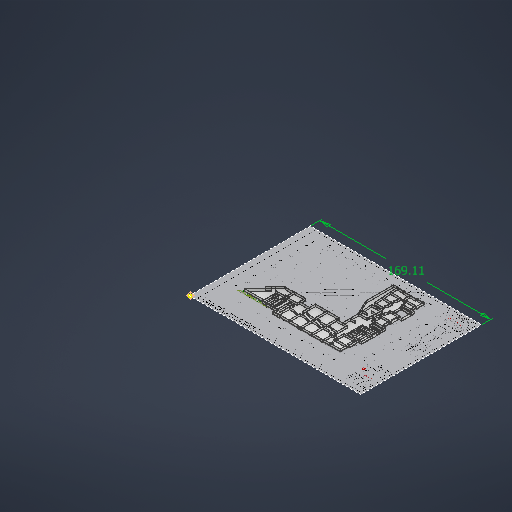
# Autodesk Inventor part: floor-6
Saved by Autodesk Inventor 2026.1 (Build 301233000, 233)
## iProperties
Created: 2025-07-25
Part Number: floor-6
Material: Generic
Document SubType Name: Modeling
Designer: diego
Density: 1 g/cm^3
Appearance: Default
Author: diego
Autodesk Inventor part; units mm, degrees
ref_plane "YZ Plane" through (0, 0, 0) normal (1, 0, 0) x (0, 1, 0)
ref_plane "XZ Plane" through (0, 0, 0) normal (0, 1, 0) x (-1, 0, 0)
ref_plane "XY Plane" through (0, 0, 0) normal (0, 0, 1) x (1, 0, 0)
sketch "Sketch1" plane through (0, 0, 0) normal (0, 1, 0) x (-1, 0, 0)
  line L0 (-169110.0554, 0) -> (0, 0) construction
  line L1 (0, 0) -> (0, -119446.8965) construction
  line L2 (0, -119446.8965) -> (-169110.0554, -119446.8965) construction
  line L3 (-169110.0554, -119446.8965) -> (-169110.0554, 0) construction
  dimension "d10" = 169110.0554
  constraints: 1 coincident, 1 horizontal, 2 other
  measures "d10" distance of L1.end L2.end
sketch "Sketch2" plane through (0, 0, 0) normal (0, 1, 0) x (-1, 0, 0)
  line L0 (-42513, -43975) -> (-42513, -44536)
  line L1 (-42513, -44536) -> (-40080, -44536)
  line L2 (-40080, -44536) -> (-36578.0094, -48027.3226)
  line L3 (-36484.618, -48120.4296) -> (-41280.5342, -52931)
  line L4 (-49108, -44536) -> (-42818, -44536)
  line L5 (-42818, -44536) -> (-42818, -43975)
  line L6 (-42818, -43975) -> (-42513, -43975)
  line L7 (-41376.4054, -52704.3063) -> (-36821.5408, -48135.524)
  line L8 (-36821.5408, -48135.524) -> (-40203.6055, -44763.7619)
  line L9 (-40203.6055, -44763.7619) -> (-42568, -44763.7619)
  line L10 (-42568, -44763.7619) -> (-49108, -44763.7619)
  line L11 (-49108, -44763.7619) -> (-49108, -44536)
  line L12 (-42513, -42019.3536) -> (-42818, -42019.3536)
  line L13 (-42818, -42019.3536) -> (-42818, -41767)
  line L14 (-42818, -41767) -> (-46373, -41767)
  line L15 (-46373, -41767) -> (-46373, -39722)
  line L16 (-46373, -39722) -> (-46111.7717, -39722)
  line L17 (-46111.7717, -39722) -> (-46111.7717, -41553)
  line L18 (-46111.7717, -41553) -> (-42818, -41553)
  line L19 (-42818, -41553) -> (-42818, -39965)
  line L20 (-42818, -39965) -> (-45192, -39965)
  line L21 (-45192, -39965) -> (-45192, -39722)
  line L22 (-45192, -39722) -> (-42818, -39722)
  line L23 (-42513, -29103) -> (-57094, -29103)
  line L24 (-42818, -39722) -> (-42818, -29418.9509)
  line L25 (-42818, -29418.9509) -> (-46077.2284, -29418.9509)
  line L26 (-46077.2284, -29418.9509) -> (-46077.2284, -37968.9509)
  line L27 (-46077.2284, -37968.9509) -> (-44184.9712, -37968.9509)
  line L28 (-44184.9712, -37968.9509) -> (-44184.9712, -38782.9509)
  line L29 (-44184.9712, -38782.9509) -> (-44428.549, -38782.9509)
  line L30 (-44428.549, -38782.9509) -> (-44428.549, -38197.9509)
  line L31 (-44428.549, -38197.9509) -> (-48923.6909, -38197.9509)
  line L32 (-48923.6909, -38197.9509) -> (-48923.6909, -37968.9509)
  line L33 (-48923.6909, -37968.9509) -> (-46371.8628, -37968.9509)
  line L34 (-46371.8628, -37968.9509) -> (-46371.8628, -29418.9509)
  line L35 (-46371.8628, -29418.9509) -> (-50128.7524, -29418.9509)
  line L36 (-50128.7524, -29418.9509) -> (-50128.7524, -30925.6566)
  line L37 (-50128.7524, -30925.6566) -> (-49818.7259, -30925.6566)
  line L38 (-49818.7259, -30925.6566) -> (-49818.7259, -42593)
  line L39 (-49818.7259, -42593) -> (-52967.8992, -42593)
  line L40 (-52967.8992, -42593) -> (-52967.8992, -42179)
  line L41 (-52967.8992, -42179) -> (-52690, -42179)
  line L42 (-52690, -42179) -> (-52690, -42386)
  line L43 (-52690, -42386) -> (-50002.0047, -42386)
  line L44 (-50002.0047, -42386) -> (-50002.0047, -41249)
  line L45 (-50002.0047, -41249) -> (-52967.8992, -41249)
  line L46 (-52967.8992, -41249) -> (-52967.8992, -40091.9961)
  line L47 (-52967.8992, -40091.9961) -> (-52690, -40091.9961)
  line L48 (-52690, -40091.9961) -> (-52690, -40645)
  line L49 (-52690, -40645) -> (-50399.2605, -40645)
  line L50 (-50399.2605, -40645) -> (-50399.2605, -31496)
  line L51 (-50399.2605, -31496) -> (-52690, -31496)
  line L52 (-52690, -31496) -> (-52690, -32210.2682)
  line L53 (-52690, -38963.0247) -> (-52690, -37818.4831)
  line L54 (-52690, -37818.4831) -> (-52989.7398, -37818.4831)
  line L55 (-52989.7398, -37818.4831) -> (-52989.7398, -38963.0247)
  line L56 (-52989.7398, -38963.0247) -> (-52690, -38963.0247)
  line L57 (-52690, -36627) -> (-52690, -35482.4583)
  line L58 (-52690, -35482.4583) -> (-52968, -35482.4583)
  line L59 (-52968, -35482.4583) -> (-52968, -36627)
  line L60 (-52968, -36627) -> (-52690, -36627)
  line L61 (-52690, -32210.2682) -> (-52981.1365, -32210.2682)
  line L62 (-52981.1365, -32210.2682) -> (-52981.1365, -30336.0449)
  line L63 (-52981.1365, -30336.0449) -> (-52690, -30336.0449)
  line L64 (-52690, -30336.0449) -> (-52690, -30925.6566)
  line L65 (-52690, -30925.6566) -> (-50348.2157, -30925.6566)
  line L66 (-50348.2157, -30925.6566) -> (-50348.2157, -29420)
  line L67 (-57093.949, -29420) -> (-57093.949, -29974)
  line L68 (-57093.949, -29974) -> (-57388.6067, -29974)
  line L69 (-57388.6067, -29974) -> (-57388.6067, -25437)
  line L70 (-57388.6067, -25437) -> (-61239, -25437)
  line L71 (-61239, -25437) -> (-61239, -30933)
  line L72 (-61239, -30933) -> (-57093.949, -30933)
  line L73 (-57093.949, -30933) -> (-57093.949, -39519)
  line L74 (-57093.949, -39519) -> (-57388.6067, -39519)
  line L75 (-57388.6067, -39519) -> (-57388.6067, -32855.7881)
  line L76 (-57388.6067, -32855.7881) -> (-60863.7297, -32855.7881)
  line L77 (-60863.7297, -32855.7881) -> (-60863.7297, -40645)
  line L78 (-60863.7297, -40645) -> (-57093.949, -40645)
  line L79 (-57093.949, -40645) -> (-57093.949, -41249)
  line L80 (-57093.949, -41249) -> (-61239, -41249)
  line L81 (-61239, -41249) -> (-61239, -42386)
  line L82 (-61239, -42386) -> (-57388.6067, -42386)
  line L83 (-57388.6067, -42386) -> (-57388.6067, -42179)
  line L84 (-57388.6067, -42179) -> (-57093.949, -42179)
  line L85 (-57093.949, -42179) -> (-57093.949, -42614.946)
  line L86 (-57093.949, -42614.946) -> (-61462, -42614.946)
  line L87 (-61462, -42614.946) -> (-61462, -37189.8355)
  line L88 (-52690, -34357) -> (-52968, -34357)
  line L89 (-52968, -34357) -> (-52968, -33212.4583)
  line L90 (-52968, -33212.4583) -> (-52690, -33212.4583)
  line L91 (-52690, -33212.4583) -> (-52690, -34357)
  line L92 (-57094, -29103) -> (-57094, -25173)
  line L93 (-106069, -25173) -> (-106069, -26456)
  line L94 (-106069, -26456) -> (-122417, -26456)
  line L95 (-122417, -26456) -> (-122417, -34675)
  line L96 (-122417, -34675) -> (-123684, -34675)
  line L97 (-123684, -34675) -> (-123684, -41595)
  line L98 (-123684, -41595) -> (-123203, -41595)
  line L99 (-123203, -41595) -> (-123203, -43594)
  line L100 (-123203, -43594) -> (-124897, -43594)
  line L101 (-124897, -43594) -> (-124897, -43216)
  line L102 (-124897, -43216) -> (-126698, -43216)
  line L103 (-126698, -43216) -> (-126698, -67258)
  line L104 (-126698, -67258) -> (-123684, -67258)
  line L105 (-123684, -83013) -> (-126698, -83013)
  line L106 (-126698, -83013) -> (-126698, -95673)
  line L107 (-123687.2606, -100717) -> (-123687.2606, -108108)
  line L108 (-126698, -95673) -> (-123687.2606, -95673)
  line L109 (-116624, -108108) -> (-116624, -107130)
  line L110 (-116624, -107130) -> (-105250, -107130)
  line L111 (-105250, -107130) -> (-105250, -108108)
  line L112 (-105250, -108108) -> (-103538, -108108)
  line L113 (-103538, -108108) -> (-103538, -107367)
  line L114 (-103538, -107367) -> (-98943, -107367)
  line L115 (-98943, -107367) -> (-98943, -108108)
  line L116 (-98943, -108108) -> (-97679, -108108)
  line L117 (-101105, -65966) -> (-109135, -65966)
  line L118 (-109135, -65966) -> (-109135, -66647)
  line L119 (-109135, -66647) -> (-108894, -66647)
  line L120 (-108894, -66647) -> (-108894, -66210)
  line L121 (-108894, -66210) -> (-101105, -66210)
  line L122 (-97919.2516, -107852) -> (-98692, -107852)
  line L123 (-98692, -107852) -> (-98692, -107130)
  line L124 (-98692, -107130) -> (-103799, -107130)
  line L125 (-103799, -107130) -> (-103799, -107852)
  line L126 (-103799, -107852) -> (-104999.5, -107852)
  line L127 (-104999.5, -107852) -> (-105019, -106553)
  line L128 (-116875, -106553) -> (-116875, -107852)
  line L129 (-116875, -107852) -> (-118103, -107852)
  line L130 (-118103, -107852) -> (-118103, -107130)
  line L131 (-118103, -107130) -> (-122208, -107130)
  line L132 (-122208, -107130) -> (-122208, -107852)
  line L133 (-122208, -107852) -> (-123443.5, -107852)
  line L134 (-123443.5, -107852) -> (-123443.5, -100932)
  line L135 (-123443.5, -100932) -> (-112664, -100932)
  line L136 (-112664, -100932) -> (-112664, -100717)
  line L137 (-112664, -100717) -> (-113079, -100717)
  line L138 (-113079, -100717) -> (-113079, -100356)
  line L139 (-113079, -100356) -> (-114086, -97996)
  line L140 (-114086, -97996) -> (-114086, -97289)
  line L141 (-114086, -97289) -> (-114324, -97289)
  line L142 (-114324, -97289) -> (-114324, -98042)
  line L143 (-114324, -98042) -> (-113315.2932, -100406)
  line L144 (-113315.2932, -100406) -> (-113315.2932, -100717)
  line L145 (-113315.2932, -100717) -> (-122760.7643, -100717)
  line L146 (-122760.7643, -100717) -> (-122760.7643, -95673)
  line L147 (-122760.7643, -95673) -> (-114324, -95673)
  line L148 (-114324, -95673) -> (-114324, -95861)
  line L149 (-114324, -95861) -> (-114086, -95861)
  line L150 (-114086, -95861) -> (-114086, -95436)
  line L151 (-114086, -95436) -> (-126429, -95436)
  line L152 (-122956.7946, -100717) -> (-123687.2606, -100717)
  line L153 (-122956.7946, -100717) -> (-122956.7946, -95673)
  line L154 (-122956.7946, -95673) -> (-123687.2606, -95673)
  line L155 (-118325, -108108) -> (-118325, -107352.6239)
  line L156 (-118325, -107352.6239) -> (-121966, -107352.6239)
  line L157 (-121966, -107352.6239) -> (-121966, -108108)
  line L158 (-123687.2606, -108108) -> (-121966, -108108)
  line L159 (-118325, -108108) -> (-116624, -108108)
  line L160 (-63603, -25173) -> (-63603, -25911)
  line L161 (-63603, -26129) -> (-63338.2659, -26129)
  line L162 (-63338.2659, -26129) -> (-63338.2659, -25437)
  line L163 (-63338.2659, -25437) -> (-61462, -25437)
  line L164 (-61462, -25437) -> (-61462, -36966.0199)
  line L165 (-61462, -36966.0199) -> (-66629.7159, -36966.0199)
  line L166 (-66629.7159, -36966.0199) -> (-69512, -35741)
  line L167 (-69512, -35741) -> (-70683, -35741)
  line L168 (-70683, -35741) -> (-70683, -36015)
  line L169 (-70683, -36015) -> (-69592, -36015)
  line L170 (-69592, -36015) -> (-66712.9965, -37189.8355)
  line L171 (-66712.9965, -37189.8355) -> (-61462, -37189.8355)
  line L172 (-81992, -26129) -> (-81992, -25437)
  line L173 (-81992, -25437) -> (-83695, -25437)
  line L174 (-83695, -25437) -> (-83695, -37189.8355)
  line L175 (-63603, -25911) -> (-81760, -25911)
  line L176 (-81760, -25911) -> (-81760, -25173)
  line L177 (-57094, -25173) -> (-63603, -25173)
  line L178 (-72110.5494, -26129) -> (-72110.5494, -37189.8355)
  line L179 (-72110.5494, -37189.8355) -> (-78291.7083, -37189.8355)
  line L180 (-78291.7083, -37189.8355) -> (-81149, -36001)
  line L181 (-81149, -36001) -> (-82278, -36001)
  line L182 (-82278, -36001) -> (-82278, -35741)
  line L183 (-82278, -35741) -> (-81124.0075, -35741)
  line L184 (-78120, -37005) -> (-72335.909, -37005)
  line L185 (-81124.0075, -35741) -> (-78120, -37005)
  line L186 (-72335.909, -37005) -> (-72335.909, -26129)
  line L187 (-63603, -26129) -> (-72110.5494, -26129)
  line L188 (-72335.909, -26129) -> (-81992, -26129)
  line L189 (-85884, -25173) -> (-85884, -25911)
  line L190 (-85884, -25911) -> (-103799, -25911)
  line L191 (-103799, -25911) -> (-103799, -25173)
  line L192 (-81760, -25173) -> (-85884, -25173)
  line L193 (-103799, -25173) -> (-106069, -25173)
  line L194 (-83942, -25437) -> (-85598, -25437)
  line L195 (-85598, -25437) -> (-85598, -26129)
  line L196 (-85598, -26129) -> (-94745, -26129)
  line L197 (-94745, -26129) -> (-94745, -37189.8355)
  line L198 (-94745, -37189.8355) -> (-100397, -37189.8355)
  line L199 (-100397, -37189.8355) -> (-103287, -36001)
  line L200 (-103287, -36001) -> (-104399.25, -36001)
  line L201 (-104399.25, -36001) -> (-104399.25, -35741)
  line L202 (-104399.25, -35741) -> (-103180.0459, -35741)
  line L203 (-103180.0459, -35741) -> (-100304.9308, -36966.0199)
  line L204 (-100304.9308, -36966.0199) -> (-94965, -36966.0199)
  line L205 (-94965, -36966.0199) -> (-94997, -26129)
  line L206 (-94997, -26129) -> (-104062, -26155.7675)
  line L207 (-104062, -26155.7675) -> (-104064.1224, -25437)
  line L208 (-104064.1224, -25437) -> (-105805, -25437)
  line L209 (-105805, -25437) -> (-105805, -37189.8355)
  line L210 (-105805, -37189.8355) -> (-107548, -37189.8355)
  line L211 (-107548, -37189.8355) -> (-107548, -36180)
  line L212 (-107548, -36180) -> (-107285, -36180)
  line L213 (-107285, -36180) -> (-107285, -36966.0199)
  line L214 (-107285, -36966.0199) -> (-106069, -36966.0199)
  line L215 (-106069, -36966.0199) -> (-106069, -34675)
  line L216 (-106069, -34675) -> (-107285, -34675)
  line L217 (-107285, -34675) -> (-107285, -35480)
  line L218 (-107285, -35480) -> (-107548, -35480)
  line L219 (-107548, -35480) -> (-107548, -34357)
  line L220 (-107548, -34357) -> (-106069, -34357)
  line L221 (-106069, -34357) -> (-106069, -26659)
  line L222 (-106069, -26659) -> (-111929, -26659)
  line L223 (-111929, -26659) -> (-111929, -27273)
  line L224 (-111929, -27273) -> (-112182, -27273)
  line L225 (-112182, -27273) -> (-112182, -26659)
  line L226 (-112182, -26659) -> (-122208, -26688.6052)
  line L227 (-122208, -26688.6052) -> (-122190.583, -32587)
  line L228 (-122190.583, -32587) -> (-111186, -32554.5052)
  line L229 (-111186, -32554.5052) -> (-111188.0744, -31852)
  line L230 (-111188.0744, -31852) -> (-112156, -29495)
  line L231 (-112156, -29495) -> (-112156, -28698)
  line L232 (-112156, -28698) -> (-111911, -28698)
  line L233 (-111911, -28698) -> (-111911, -29394.3883)
  line L234 (-111911, -29394.3883) -> (-110901.7572, -31852)
  line L235 (-110901.7572, -31852) -> (-110901.7572, -32841)
  line L236 (-110901.7572, -32841) -> (-112262, -32841)
  line L237 (-83695, -37189.8355) -> (-89336, -37189.8355)
  line L238 (-89336, -37189.8355) -> (-92207, -36001)
  line L239 (-92207, -36001) -> (-93305, -36001)
  line L240 (-93305, -36001) -> (-93305, -35741)
  line L241 (-93305, -35741) -> (-92253.8679, -35741)
  line L242 (-92253.8679, -35741) -> (-89256.377, -36982.2133)
  line L243 (-89256.377, -36982.2133) -> (-83942, -36982.2133)
  line L244 (-83942, -36982.2133) -> (-83942, -25437)
  line L245 (-112262, -32841) -> (-112262, -33787)
  line L246 (-112262, -33787) -> (-112536, -33787)
  line L247 (-112536, -33787) -> (-112536, -32841)
  line L248 (-112536, -32841) -> (-122190.583, -32841)
  line L249 (-122190.583, -32841) -> (-122190.583, -34675)
  line L250 (-122190.583, -34675) -> (-121476, -34675)
  line L251 (-121476, -34675) -> (-121476, -39488)
  line L252 (-121476, -39488) -> (-121764, -39488)
  line L253 (-121764, -39488) -> (-121764, -34918.5)
  line L254 (-121764, -34918.5) -> (-123443.5, -34918.5)
  line L255 (-123443.5, -34918.5) -> (-123443.5, -41358)
  line L256 (-123443.5, -41358) -> (-121764, -41358)
  line L257 (-121764, -41358) -> (-121764, -40372)
  line L258 (-121764, -40372) -> (-121476, -40372)
  line L259 (-121476, -40372) -> (-121476, -41358)
  line L260 (-121476, -41358) -> (-111188.0744, -41358)
  line L261 (-111188.0744, -41358) -> (-111188.0744, -34239)
  line L262 (-111188.0744, -34239) -> (-110901.7572, -34239)
  line L263 (-110901.7572, -34239) -> (-110901.7572, -41595)
  line L264 (-110901.7572, -41595) -> (-112451.0512, -41595)
  line L265 (-42513, -30862) -> (-23317, -30862)
  line L266 (-23317, -30862) -> (-33849.7934, -41426.9769)
  line L267 (-33849.7934, -41426.9769) -> (-31824.5142, -43446.0866)
  line L268 (-31824.5142, -43446.0866) -> (-36484.618, -48120.4296)
  line L269 (-36578.0094, -48027.3226) -> (-35002.7605, -46447.2604)
  line L270 (-35002.7605, -46447.2604) -> (-36065.2829, -45387.9747)
  line L271 (-36065.2829, -45387.9747) -> (-35971.7729, -45294.1789)
  line L272 (-35971.7729, -45294.1789) -> (-34909.2504, -46353.4646)
  line L273 (-34909.2504, -46353.4646) -> (-32010.5516, -43445.9087)
  line L274 (-32010.5516, -43445.9087) -> (-33961.064, -41501.3379)
  line L275 (-33961.064, -41501.3379) -> (-36859.7629, -44408.8939)
  line L276 (-36859.7629, -44408.8939) -> (-36940.9533, -44327.9509)
  line L277 (-36940.9533, -44327.9509) -> (-23666.8941, -31013.3321)
  line L278 (-23666.8941, -31013.3321) -> (-42513, -31013.3321)
  line L279 (-42513, -42019.3536) -> (-42513, -31013.3321)
  line L280 (-42513, -30862) -> (-42513, -29103)
  line L281 (-110901.7572, -106553) -> (-110920, -100326)
  line L282 (-110920, -100326) -> (-110607, -100325.083)
  line L283 (-110607, -100325.083) -> (-110607.7063, -100084)
  line L284 (-110607.7063, -100084) -> (-111158, -100085.6122)
  line L285 (-111158, -100085.6122) -> (-111156.2089, -100697)
  line L286 (-111156.2089, -100697) -> (-111257, -100697)
  line L287 (-111257, -100697) -> (-111257, -100932)
  line L288 (-111257, -100932) -> (-111155.5204, -100932)
  line L289 (-111155.5204, -100932) -> (-111155.5204, -106553)
  line L290 (-105019, -106553) -> (-110901.7572, -106553)
  line L291 (-111155.5204, -106553) -> (-116875, -106553)
  line L292 (-98495.0852, -100325.083) -> (-109188, -100325.083)
  line L293 (-109188, -100325.083) -> (-109188, -100085.6122)
  line L294 (-109188, -100085.6122) -> (-108600, -100085.6122)
  line L295 (-108600, -100085.6122) -> (-108600, -96895)
  line L296 (-108600, -96895) -> (-107568, -94466)
  line L297 (-107568, -94466) -> (-107568, -93705)
  line L298 (-107568, -93705) -> (-107345, -93705)
  line L299 (-107345, -93705) -> (-107345, -94538)
  line L300 (-107345, -94538) -> (-108305, -96895)
  line L301 (-108305, -96895) -> (-108331, -100085.6122)
  line L302 (-108331, -100085.6122) -> (-98513.4055, -100085.6122)
  line L303 (-98495.0852, -100325.083) -> (-97919.2516, -107852)
  line L304 (-107568, -92277) -> (-107568, -91875)
  line L305 (-107568, -91875) -> (-108600, -91875)
  line L306 (-107568, -92277) -> (-107345, -92277)
  line L307 (-107345, -92277) -> (-107345, -91875)
  line L308 (-107345, -91875) -> (-99141.5441, -91875)
  line L309 (-108600, -91875) -> (-108600, -88430)
  line L310 (-108600, -88430) -> (-107589, -86050)
  line L311 (-107589, -86050) -> (-107589, -85277)
  line L312 (-107589, -85277) -> (-107320, -85277)
  line L313 (-107320, -85277) -> (-107320, -86119)
  line L314 (-107320, -86119) -> (-108331, -88499)
  line L315 (-108331, -88499) -> (-108331, -91605)
  line L316 (-108331, -91605) -> (-99162.1999, -91605)
  line L317 (-99141.5441, -91875) -> (-98513.4055, -100085.6122)
  line L318 (-107589, -83870) -> (-107589, -83174)
  line L319 (-107589, -83174) -> (-99586.5321, -83174)
  line L320 (-107589, -83870) -> (-107320, -83870)
  line L321 (-107320, -83870) -> (-107320, -83453)
  line L322 (-107320, -83453) -> (-99785.8544, -83453)
  line L323 (-99785.8544, -83453) -> (-99162.1999, -91605)
  line L324 (-99807.1989, -80289.5893) -> (-104399.25, -80289.5893)
  line L325 (-104399.25, -80289.5893) -> (-104399.25, -80015)
  line L326 (-104399.25, -80015) -> (-100048.8726, -80015)
  line L327 (-97696.9018, -107874) -> (-99586.5321, -83174)
  line L328 (-99807.1989, -80289.5893) -> (-100887.6228, -66167)
  line L329 (-105250, -80289.5893) -> (-110165.0407, -80289.5893)
  line L330 (-110165.0407, -80289.5893) -> (-110165.0407, -71171.3975)
  line L331 (-105250, -80289.5893) -> (-105250, -80015.4686)
  line L332 (-105250, -80015.4686) -> (-109894.9237, -80015.4686)
  line L333 (-109894.9237, -80015.4686) -> (-109894.9237, -74759.4686)
  line L334 (-109894.9237, -74759.4686) -> (-104830.9237, -74759.4686)
  line L335 (-104830.9237, -74759.4686) -> (-104830.9237, -74502.4686)
  line L336 (-104830.9237, -74502.4686) -> (-109894.9237, -74502.4686)
  line L337 (-109894.9237, -74502.4686) -> (-109894.9237, -71209.4686)
  line L338 (-109894.9237, -71209.4686) -> (-108894, -68909)
  line L339 (-108894, -68909) -> (-108894, -68054)
  line L340 (-108894, -68054) -> (-109135, -68054)
  line L341 (-109135, -68054) -> (-109135, -68804.0078)
  line L342 (-109135, -68804.0078) -> (-110165.0407, -71171.3975)
  line L343 (-100774.965, -70524) -> (-104878, -70524)
  line L344 (-104878, -70524) -> (-104878, -70370)
  line L345 (-104878, -70370) -> (-100786.7465, -70370)
  line L346 (-101105, -66210) -> (-100786.7465, -70370)
  line L347 (-100774.965, -70524) -> (-100048.8726, -80015)
  line L348 (-97679, -108108) -> (-93722, -108108)
  line L349 (-93722, -108108) -> (-93722, -80393)
  line L350 (-93722, -80393) -> (-100641, -65966)
  line L351 (-100641, -65966) -> (-100903, -65966)
  line L352 (-100887.6228, -66167) -> (-100772, -66167)
  line L353 (-100772, -66167) -> (-93907, -80481.7236)
  line L354 (-93907, -80481.7236) -> (-93907, -107874)
  line L355 (-93907, -107874) -> (-97696.9018, -107874)
  line L356 (-100903, -65966) -> (-100903, -50169)
  line L357 (-100903, -50169) -> (-94997, -50169)
  line L358 (-94997, -50169) -> (-94997, -52931)
  line L359 (-94997, -52931) -> (-71582, -52931)
  line L360 (-71582, -40113.47) -> (-72793, -40113.47)
  line L361 (-72793, -40113.47) -> (-72793, -40343)
  line L362 (-72793, -40343) -> (-71827, -40343)
  line L363 (-71827, -40343) -> (-71827, -52704)
  line L364 (-71827, -52704) -> (-83159, -52704)
  line L365 (-83159, -52704) -> (-83159, -40343)
  line L366 (-83159, -40343) -> (-78423.0736, -40343)
  line L367 (-78423.0736, -40343) -> (-75441, -41595)
  line L368 (-75441, -41595) -> (-74219, -41595)
  line L369 (-74219, -41595) -> (-74219, -41358)
  line L370 (-74219, -41358) -> (-75341.4974, -41358)
  line L371 (-75341.4974, -41358) -> (-78395.015, -40113.47)
  line L372 (-78395.015, -40113.47) -> (-83853, -40113.47)
  line L373 (-83853, -40113.47) -> (-83853, -40343)
  line L374 (-83853, -40343) -> (-83404, -40343)
  line L375 (-83404, -40343) -> (-83404, -52704)
  line L376 (-83404, -52704) -> (-94745, -52704)
  line L377 (-94745, -52704) -> (-94779, -40343)
  line L378 (-94779, -40343) -> (-89442, -40343)
  line L379 (-89442, -40343) -> (-86495, -41595)
  line L380 (-86495, -41595) -> (-85268, -41595)
  line L381 (-85268, -41595) -> (-85268, -41358)
  line L382 (-85268, -41358) -> (-86394.3132, -41358)
  line L383 (-86394.3132, -41358) -> (-89341.3132, -40106)
  line L384 (-89341.3132, -40106) -> (-94997, -40106)
  line L385 (-94997, -40106) -> (-94997, -49890)
  line L386 (-94997, -49890) -> (-105805, -49890)
  line L387 (-105805, -49890) -> (-105805, -40373.328)
  line L388 (-105805, -40373.328) -> (-100543, -40373.328)
  line L389 (-100543, -40373.328) -> (-97679, -41553)
  line L390 (-97679, -41553) -> (-96403, -41553)
  line L391 (-96403, -41553) -> (-96403, -41358)
  line L392 (-96403, -41358) -> (-97598.6802, -41358)
  line L393 (-97598.6802, -41358) -> (-100543, -40145.2445)
  line L394 (-100543, -40145.2445) -> (-106069, -40106)
  line L395 (-106069, -40106) -> (-106069, -50169)
  line L396 (-106069, -50169) -> (-101227.9016, -50169)
  line L397 (-101227.9016, -50169) -> (-101227.9016, -57549.3186)
  line L398 (-101227.9016, -57549.3186) -> (-105885, -57549.3186)
  line L399 (-105885, -57549.3186) -> (-105885, -57825)
  line L400 (-104934.5612, -57825) -> (-101105, -57825)
  line L401 (-101105, -57825) -> (-101105, -65966)
  line L402 (-105885, -57825) -> (-105885, -58561)
  line L403 (-105885, -58561) -> (-104934.5612, -58561)
  line L404 (-104934.5612, -58561) -> (-104934.5612, -57825)
  line L405 (-123050.5, -41595) -> (-123050.5, -43594)
  line L406 (-123050.5, -43594) -> (-119763, -43594)
  line L407 (-119763, -43594) -> (-119763, -43182)
  line L408 (-119763, -43182) -> (-118228, -43182)
  line L409 (-118228, -43182) -> (-118228, -42477)
  line L410 (-118228, -42477) -> (-118038.0288, -42477)
  line L411 (-118038.0288, -42477) -> (-118038.0288, -43182)
  line L412 (-123050.5, -41595) -> (-112579.6322, -41595)
  line L413 (-112579.6322, -41595) -> (-112579.6322, -43243.7905)
  line L414 (-112579.6322, -43243.7905) -> (-112451.0512, -43243.7905)
  line L415 (-112451.0512, -43243.7905) -> (-112451.0512, -41595)
  line L416 (-118038.0288, -43182) -> (-117947, -43182)
  line L417 (-117947, -43182) -> (-117947, -44255.5)
  line L418 (-117947, -44255.5) -> (-112451.0512, -44255.5)
  line L419 (-112451.0512, -44255.5) -> (-112451.0512, -44372)
  line L420 (-112451.0512, -44372) -> (-117947, -44372)
  line L421 (-117947, -44372) -> (-117947, -46949)
  line L422 (-117947, -46949) -> (-112579.6322, -46949)
  line L423 (-112579.6322, -46949) -> (-112579.6322, -45293.9193)
  line L424 (-112579.6322, -45293.9193) -> (-112451.0512, -45293.9193)
  line L425 (-112451.0512, -45293.9193) -> (-112451.0512, -48854)
  line L426 (-112451.0512, -48854) -> (-112579.6322, -48854)
  line L427 (-112579.6322, -48854) -> (-112579.6322, -47073.9597)
  line L428 (-112579.6322, -47073.9597) -> (-117947, -47073.9597)
  line L429 (-117947, -47073.9597) -> (-117947, -49890)
  line L430 (-117947, -49890) -> (-112601, -49890)
  line L431 (-112601, -49890) -> (-112601, -49764)
  line L432 (-112601, -49764) -> (-112451.0512, -49764)
  line L433 (-112451.0512, -49764) -> (-112451.0512, -52454)
  line L434 (-112451.0512, -52454) -> (-112664, -52454)
  line L435 (-112664, -52454) -> (-112664, -50169)
  line L436 (-112664, -50169) -> (-115725, -50169)
  line L437 (-115725, -50169) -> (-115725, -52207)
  line L438 (-115725, -52207) -> (-113582.5, -52207)
  line L439 (-113582.5, -52207) -> (-113582.5, -52454)
  line L440 (-113582.5, -52454) -> (-117061, -52454)
  line L441 (-117061, -52454) -> (-117061, -52207)
  line L442 (-117061, -52207) -> (-115936, -52207)
  line L443 (-115936, -52207) -> (-115936, -50169)
  line L444 (-115936, -50169) -> (-117947, -50169)
  line L445 (-117947, -52454) -> (-121189, -52454)
  line L446 (-121189, -52454) -> (-121189, -52207)
  line L447 (-121189, -52207) -> (-118228, -52207)
  line L448 (-118228, -52207) -> (-118228, -43816)
  line L449 (-118228, -43816) -> (-122177.9121, -43816)
  line L450 (-122177.9121, -43816) -> (-122177.9121, -52207)
  line L451 (-122177.9121, -52207) -> (-122037, -52207)
  line L452 (-122037, -52207) -> (-122037, -52454)
  line L453 (-122037, -52454) -> (-125405, -52454)
  line L454 (-125405, -52454) -> (-125405, -52207)
  line L455 (-125405, -52207) -> (-122478, -52207)
  line L456 (-122478, -52207) -> (-122478, -43816)
  line L457 (-122478, -43816) -> (-126429, -43816)
  line L458 (-126429, -43816) -> (-126429, -52207)
  line L459 (-126429, -52207) -> (-126281, -52207)
  line L460 (-126281, -52207) -> (-126281, -52454)
  line L461 (-126281, -52454) -> (-126497, -52454)
  line L462 (-126497, -52454) -> (-126497, -53869.0099)
  line L463 (-117947, -52454) -> (-117947, -50169)
  line L464 (-126497, -53869.0099) -> (-116983.362, -53869.0099)
  line L465 (-116983.362, -53869.0099) -> (-116983.362, -54144)
  line L466 (-116983.362, -54144) -> (-117599, -54144)
  line L467 (-117599, -54144) -> (-117599, -58067.5)
  line L468 (-117599, -58067.5) -> (-116836.4153, -58067.5)
  line L469 (-116836.4153, -58067.5) -> (-116836.4153, -58436)
  line L470 (-116836.4153, -58436) -> (-116052.1429, -58436)
  line L471 (-116052.1429, -58436) -> (-116052.1429, -53869.0099)
  line L472 (-116052.1429, -53869.0099) -> (-115784.155, -53869.0099)
  line L473 (-115784.155, -53869.0099) -> (-115784.155, -57202.8544)
  line L474 (-115784.155, -57202.8544) -> (-114413, -57202.8544)
  line L475 (-114413, -57202.8544) -> (-114413, -54144)
  line L476 (-114413, -54144) -> (-114841, -54144)
  line L477 (-114841, -54144) -> (-114841, -53869.0099)
  line L478 (-114841, -53869.0099) -> (-113620.836, -53869.0099)
  line L479 (-113620.836, -53869.0099) -> (-113620.836, -54144)
  line L480 (-113620.836, -54144) -> (-114135.9834, -54144)
  line L481 (-114135.9834, -54144) -> (-114135.9834, -57202.8544)
  line L482 (-114135.9834, -57202.8544) -> (-112731, -57202.8544)
  line L483 (-112731, -57202.8544) -> (-112731, -53869.0099)
  line L484 (-112731, -53869.0099) -> (-112451.0512, -53869.0099)
  line L485 (-112451.0512, -53869.0099) -> (-112451.0512, -58716)
  line L486 (-112451.0512, -58716) -> (-112731, -58716)
  line L487 (-112731, -58716) -> (-112731, -57439.6649)
  line L488 (-112731, -57439.6649) -> (-115784.155, -57439.6649)
  line L489 (-115784.155, -57439.6649) -> (-115784.155, -58716)
  line L490 (-117112.7606, -58716) -> (-117112.7606, -58365)
  line L491 (-117112.7606, -58365) -> (-117865.6619, -58365)
  line L492 (-117865.6619, -58365) -> (-117865.6619, -54144)
  line L493 (-117112.7606, -58716) -> (-115784.155, -58716)
  line L494 (-117865.6619, -54144) -> (-119879, -54144)
  line L495 (-119879, -54144) -> (-119879, -54464)
  line L496 (-119879, -54464) -> (-125684, -54464)
  line L497 (-125684, -54464) -> (-125684, -57779.4009)
  line L498 (-125684, -57779.4009) -> (-119879, -57779.4009)
  line L499 (-119879, -57779.4009) -> (-119879, -58077.8324)
  line L500 (-119879, -58077.8324) -> (-118995.5, -58077.8324)
  line L501 (-118995.5, -58077.8324) -> (-118995.5, -58365)
  line L502 (-118995.5, -58365) -> (-126389, -58365)
  line L503 (-126389, -58365) -> (-126389, -61540)
  line L504 (-116152, -61540) -> (-116152, -64478)
  line L505 (-116152, -64478) -> (-126389, -64478)
  line L506 (-126389, -64478) -> (-126389, -67028.752)
  line L507 (-126389, -67028.752) -> (-116423.3415, -67028.752)
  line L508 (-116423.3415, -67028.752) -> (-116423.3415, -65347)
  line L509 (-116423.3415, -65347) -> (-116152, -65347)
  line L510 (-116152, -65347) -> (-116152, -66131.3665)
  line L511 (-116152, -66131.3665) -> (-115970.4211, -66131.3665)
  line L512 (-115970.4211, -66131.3665) -> (-115970.4211, -67028.752)
  line L513 (-115970.4211, -67028.752) -> (-113052.3248, -67028.752)
  line L514 (-113052.3248, -67028.752) -> (-113052.3248, -70046.7807)
  line L515 (-118122.8418, -61841) -> (-118122.8418, -61540)
  line L516 (-119307.3837, -61841) -> (-119307.3837, -61540)
  line L517 (-119307.3837, -61841) -> (-118122.8418, -61841)
  line L518 (-120427.729, -61540) -> (-120427.729, -61841)
  line L519 (-120427.729, -61841) -> (-121612.271, -61841)
  line L520 (-121612.271, -61841) -> (-121612.271, -61540)
  line L521 (-122741.4227, -61540) -> (-122741.4227, -61841)
  line L522 (-122741.4227, -61841) -> (-123941.5, -61841)
  line L523 (-123941.5, -61841) -> (-123941.5, -61540)
  line L524 (-125051, -61540) -> (-125051, -61841)
  line L525 (-125051, -61841) -> (-126389, -61841)
  line L526 (-126389, -61841) -> (-126389, -64112.4249)
  line L527 (-126389, -64112.4249) -> (-116498.5, -64193)
  line L528 (-116498.5, -64193) -> (-116498.5, -61841)
  line L529 (-116498.5, -61841) -> (-117026.6444, -61841)
  line L530 (-117026.6444, -61841) -> (-117026.6444, -61540)
  line L531 (-117026.6444, -61540) -> (-116152, -61540)
  line L532 (-113052.3248, -70046.7807) -> (-114086, -72414.0457)
  line L533 (-114086, -72414.0457) -> (-114086, -73179.5)
  line L534 (-114086, -73179.5) -> (-114324, -73179.5)
  line L535 (-114324, -73179.5) -> (-114324, -72414.0457)
  line L536 (-114324, -72414.0457) -> (-113315.2932, -70046.7807)
  line L537 (-113315.2932, -70046.7807) -> (-113315.2932, -67258)
  line L538 (-113315.2932, -67258) -> (-123443.5, -67258)
  line L539 (-123443.5, -67258) -> (-123443.5, -68429.0039)
  line L540 (-123443.5, -68429.0039) -> (-122692.25, -68429.0039)
  line L541 (-122692.25, -68429.0039) -> (-122692.25, -73832)
  line L542 (-122692.25, -73832) -> (-123443.5, -73832)
  line L543 (-123443.5, -73832) -> (-123443.5, -75039)
  line L544 (-123443.5, -75039) -> (-114324, -75039)
  line L545 (-114324, -75039) -> (-114324, -74576)
  line L546 (-114324, -74576) -> (-114086, -74576)
  line L547 (-114086, -74576) -> (-114086, -75039)
  line L548 (-114086, -75039) -> (-113052.3248, -75039)
  line L549 (-113052.3248, -75039) -> (-113052.3248, -79034)
  line L550 (-113052.3248, -79034) -> (-114086, -81433)
  line L551 (-114086, -81433) -> (-114086, -82160)
  line L552 (-114086, -82160) -> (-114324, -82160)
  line L553 (-114324, -82160) -> (-114324, -81433)
  line L554 (-114324, -81433) -> (-113315.2932, -78995)
  line L555 (-113315.2932, -78995) -> (-113315.2932, -75269.5)
  line L556 (-113315.2932, -75269.5) -> (-123443.5, -75269.5)
  line L557 (-123443.5, -75269.5) -> (-123443.5, -76415)
  line L558 (-123443.5, -76415) -> (-122692.25, -76415)
  line L559 (-122692.25, -76415) -> (-122692.25, -81841)
  line L560 (-122692.25, -81841) -> (-123443.5, -81841)
  line L561 (-123443.5, -81841) -> (-123443.5, -84113)
  line L562 (-123443.5, -84113) -> (-114324, -84113)
  line L563 (-114324, -84113) -> (-114324, -83600.3172)
  line L564 (-114324, -83600.3172) -> (-114086, -83600.3172)
  line L565 (-114086, -83600.3172) -> (-114086, -84346.2118)
  line L566 (-123687.2606, -84392.2053) -> (-123687.2606, -83291)
  line L567 (-123687.2606, -83291) -> (-126429, -83291)
  line L568 (-126429, -83291) -> (-126429, -92277)
  line L569 (-126429, -92277) -> (-116727.2925, -92277)
  line L570 (-116727.2925, -92277) -> (-116727.2925, -84392.2053)
  line L571 (-116451.6113, -84346.2118) -> (-116451.6113, -91777.0235)
  line L572 (-116451.6113, -91777.0235) -> (-115961.3062, -91777.0235)
  line L573 (-115961.3062, -91777.0235) -> (-115961.3062, -92762.9765)
  line L574 (-115961.3062, -92762.9765) -> (-116982, -92762.9765)
  line L575 (-116982, -92762.9765) -> (-116982, -92535)
  line L576 (-116982, -92535) -> (-118065.6086, -92535)
  line L577 (-118065.6086, -92535) -> (-118065.6086, -94322.3301)
  line L578 (-118065.6086, -94322.3301) -> (-118297.4201, -94322.3301)
  line L579 (-118297.4201, -94322.3301) -> (-118297.4201, -92535)
  line L580 (-118297.4201, -92535) -> (-126429, -92535)
  line L581 (-126429, -92535) -> (-126429, -95436)
  line L582 (-114086, -84346.2118) -> (-116451.6113, -84346.2118)
  line L583 (-116727.2925, -84392.2053) -> (-123687.2606, -84392.2053)
  line L584 (-122956.7946, -73587) -> (-122956.7946, -68652.3903)
  line L585 (-122956.7946, -68652.3903) -> (-123684, -68652.3903)
  line L586 (-122956.7946, -73587) -> (-123684, -73587)
  line L587 (-123684, -67258) -> (-123684, -68652.3903)
  line L588 (-123684, -73587) -> (-123684, -83013)
  line L589 (-61815.1123, -47084) -> (-71582, -47084)
  line L590 (-71582, -46949) -> (-61811, -46988)
  line L591 (-61811, -46988) -> (-61811, -44536)
  line L592 (-71582, -52931) -> (-71582, -47084)
  line L593 (-71582, -46949) -> (-71582, -40113.47)
  line L594 (-36578.0094, -48027.3226) -> (-36484.618, -48120.4296)
  line L595 (-49355, -52704.3063) -> (-49355, -52207)
  line L596 (-49355, -52207) -> (-42110, -52207)
  line L597 (-42110, -52207) -> (-42110, -52704.3063)
  line L598 (-42330, -52931) -> (-42330, -52397)
  line L599 (-42330, -52397) -> (-49108, -52397)
  line L600 (-49108, -52397) -> (-49108, -52931)
  line L601 (-41280.5342, -52931) -> (-42330, -52931)
  line L602 (-42110, -52704.3063) -> (-41376.4054, -52704.3063)
  line L603 (-49108, -52931) -> (-61815.1123, -52931)
  line L604 (-61815.1123, -52931) -> (-61815.1123, -47084)
  line L605 (-61811, -44536) -> (-52152, -44536)
  line L606 (-52152, -44536) -> (-52152, -44763.7619)
  line L607 (-52152, -44763.7619) -> (-61561.3369, -44763.7619)
  line L608 (-61561.3369, -44763.7619) -> (-61561.3369, -52704.3063)
  line L609 (-61561.3369, -52704.3063) -> (-50756.8092, -52704.3063)
  line L610 (-50756.8092, -52704.3063) -> (-50756.8092, -46121.4597)
  line L611 (-50756.8092, -46121.4597) -> (-52544, -46121.4597)
  line L612 (-52544, -46121.4597) -> (-52544, -45885.5861)
  line L613 (-52544, -45885.5861) -> (-50756.8092, -45885.5861)
  line L614 (-50756.8092, -45885.5861) -> (-50756.8092, -44536)
  line L615 (-50507.7253, -44536) -> (-50507.7253, -45885.5861)
  line L616 (-50507.7253, -45885.5861) -> (-48710, -45885.5861)
  line L617 (-48710, -45885.5861) -> (-48710, -46121.4597)
  line L618 (-48710, -46121.4597) -> (-50507.7253, -46121.4597)
  line L619 (-50507.7253, -52704.3063) -> (-49355, -52704.3063)
  line L620 (-50507.7253, -46121.4597) -> (-50507.7253, -52704.3063)
  line L621 (-50507.7253, -44536) -> (-50756.8092, -44536)
  line L622 (-119307.3837, -61540) -> (-118122.8418, -61540)
  line L623 (-121612.271, -61540) -> (-120427.729, -61540)
  line L624 (-126389, -61540) -> (-125051, -61540)
  line L625 (-123941.5, -61540) -> (-122741.4227, -61540)
  line L626 (-52690, -29420) -> (-52690, -29637.8026)
  line L627 (-52690, -29637.8026) -> (-52968, -29637.8026)
  line L628 (-52968, -29637.8026) -> (-52968, -29420)
  line L629 (-50348.2157, -29420) -> (-52690, -29420)
  line L630 (-52968, -29420) -> (-57093.949, -29420)
  point P0 (0, 0)
  constraints: 1263 end point, 413 perpendicular, 176 point on line, 52 parallel, 50 vertical, 49 horizontal, 8 collinear, 3 equal length, 1 other
extrude "Walls" add sketch "Sketch2" along normal blind 2300
extrude "Extrusion5" add sketch "Sketch2" along normal blind 300 contours L6 L5 L4 L11 L10 L9 L8 L7 L602 L597 L596 L595 L619 L620 L618 L617 L616 L615 L621 L614 L613 L612 L611 L610 L609 L608 L607 L606 L605 L591 L590 L593 L360 L361 L362 L363 L364 L365 L366 L367 L368 L369 L370 L371 L372 L373 L374 L375 L376 L377 L378 L379 L380 L381 L382 L383 L384 L385 L386 L387 L388 L389 L390 L391 L392 L393 L394 L395 L396 L397 L398 L399 L402 L403 L404 L400 L401 L117 L118 L119 L120 L121 L346 L345 L344 L343 L347 L326 L325 L324 L328 L352 L353 L354 L355 L327 L319 L318 L320 L321 L322 L323 L316 L315 L314 L313 L312 L311 L310 L309 L305 L304 L306 L307 L308 L317 L302 L301 L300 L299 L298 L297 L296 L295 L294 L293 L292 L303 L122 L123 L124 L125 L126 L127 L290 L281 L282 L283 L284 L285 L286 L287 L288 L289 L291 L128 L129 L130 L131 L132 L133 L134 L135 L136 L137 L138 L139 L140 L141 L142 L143 L144 L145 L146 L147 L148 L149 L150 L151 L581 L580 L579 L578 L577 L576 L575 L574 L573 L572 L571 L582 L565 L564 L563 L562 L561 L560 L559 L558 L557 L556 L555 L554 L553 L552 L551 L550 L549 L548 L547 L546 L545 L544 L543 L542 L541 L540 L539 L538 L537 L536 L535 L534 L533 L532 L514 L513 L512 L511 L510 L509 L508 L507 L506 L505 L504 L531 L530 L529 L528 L527 L526 L525 L524 L624 L503 L502 L501 L500 L499 L498 L497 L496 L495 L494 L492 L491 L490 L493 L489 L488 L487 L486 L485 L484 L483 L482 L481 L480 L479 L478 L477 L476 L475 L474 L473 L472 L471 L470 L469 L468 L467 L466 L465 L464 L462 L461 L460 L459 L458 L457 L456 L455 L454 L453 L452 L451 L450 L449 L448 L447 L446 L445 L463 L444 L443 L442 L441 L440 L439 L438 L437 L436 L435 L434 L433 L432 L431 L430 L429 L428 L427 L426 L425 L424 L423 L422 L421 L420 L419 L418 L417 L416 L411 L410 L409 L408 L407 L406 L405 L412 L413 L414 L415 L264 L263 L262 L261 L260 L259 L258 L257 L256 L255 L254 L253 L252 L251 L250 L249 L248 L247 L246 L245 L236 L235 L234 L233 L232 L231 L230 L229 L228 L227 L226 L225 L224 L223 L222 L221 L220 L219 L218 L217 L216 L215 L214 L213 L212 L211 L210 L209 L208 L207 L206 L205 L204 L203 L202 L201 L200 L199 L198 L197 L196 L195 L194 L244 L243 L242 L241 L240 L239 L238 L237 L174 L173 L172 L188 L186 L184 L185 L183 L182 L181 L180 L179 L178 L187 L161 L162 L163 L164 L165 L166 L167 L168 L169 L170 L171 L87 L86 L85 L84 L83 L82 L81 L80 L79 L78 L77 L76 L75 L74 L73 L72 L71 L70 L69 L68 L67 L630 L628 L627 L626 L629 L66 L65 L64 L63 L62 L61 L52 L51 L50 L49 L48 L47 L46 L45 L44 L43 L42 L41 L40 L39 L38 L37 L36 L35 L34 L33 L32 L31 L30 L29 L28 L27 L26 L25 L24 L22 L21 L20 L19 L18 L17 L16 L15 L14 L13 L12 L279 L278 L277 L276 L275 L274 L273 L272 L271 L270 L269 L2 L1 L0
body "Solid3"
